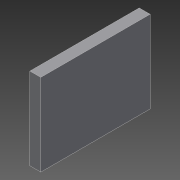
# Autodesk Inventor part: trackballL
Saved by Autodesk Inventor 2018 (Build 220112000, 112)
## iProperties
Created: 2018-06-15
Part Number: trackballL
Material: 一般
Document SubType Name: Sheet Metal
Designer: NaMACHAN
Density: 1 g/cm^3
Sheet Metal Rule: Default
Appearance: 既定
Author: NaMACHAN
Autodesk Inventor part; units mm, degrees
ref_plane "YZ Plane" through (0, 0, 0) normal (1, 0, 0) x (0, 1, 0)
ref_plane "XZ Plane" through (0, 0, 0) normal (0, 1, 0) x (-1, 0, 0)
ref_plane "XY Plane" through (0, 0, 0) normal (0, 0, 1) x (1, 0, 0)
sketch "スケッチ1" plane through (0, 0, 0) normal (1, 0, 0) x (0, 1, 0)
  line L0 (-10, -10) -> (10, -10)
  line L1 (10, -10) -> (10, 10)
  line L2 (10, 10) -> (-10, 10)
  line L3 (-10, 10) -> (-10, -10)
  line L4 (-10, -10) -> (10, 10) construction
  line L5 (10, -10) -> (-10, 10) construction
  point P0 (0, 0)
  dimension "d0" = 20
  dimension "d1" = 20
  measures "d0" distance of L2.end L1.end
  measures "d1" distance of L1.end L0.end
extrude "プレート1" add sketch "スケッチ1" along normal blind 2
sketch "スケッチ2" plane through (4, 12, 10) normal (0, 1, 0) x (-1, 0, 0)
  line L0 (0, -20) -> (0, 0)
  line L1 (0, 0) -> (-21, 0)
  line L2 (-21, 0) -> (-21, -20)
  line L3 (-21, -20) -> (0, -20)
  constraints: 6 end point, 1 horizontal, 1 perpendicular, 1 vertical
edge flange "フランジ1" height 25 angle 90 thickness 2 bend radius 2 thickness toward (0, 1, 0) relief straight relief width 2 relief depth 1 edges at (2, 10, 0) wall of the first edge with corners at (4, 12, -10) (4, 12, 10) (25, 12, 10) (25, 12, -10)
bend "曲げ1"
corner "コーナー1"
sketch "スケッチ3" plane through (0, 0, 0) normal (-1, 0, 0) x (0, 0, 1)
  line L0 (-7.5, 6) -> (-7.5, -6)
  arc A0 (-7.5, -6) -> (-4.5, -6) centre (-6, -6) ccw
  line L1 (-4.5, -6) -> (-4.5, 6)
  arc A1 (-4.5, 6) -> (-7.5, 6) centre (-6, 6) ccw
  line L2 (4.5, 6) -> (4.5, -6)
  arc A2 (4.5, -6) -> (7.5, -6) centre (6, -6) ccw
  line L3 (7.5, -6) -> (7.5, 6)
  arc A3 (7.5, 6) -> (4.5, 6) centre (6, 6) ccw
  line L4 (-10, -10) -> (-10, 10) projected
  line L5 (10, 10) -> (10, -10) projected
  line L6 (10, -10) -> (-10, -10) projected
  line L7 (-10, 10) -> (10, 10) projected
  point P0 (0, 0)
  dimension "d13" = 4
  dimension "d14" = 4
  dimension "d15" = 1.5
  dimension "d16" = 1.5
  dimension "d17" = 4
  dimension "d18" = 4
  dimension "d19" = 4
  dimension "d20" = 4
  constraints: 8 end point, 8 point on circle, 8 tangent, 4 centre point, 2 parallel, 2 vertical
  measures "d13" distance from line of L4 A1.centre
  measures "d14" distance from line of L5 A3.centre
  measures "d15" radius of A1
  measures "d16" radius of A3
  measures "d17" distance from line of L6 A0.centre
  measures "d18" distance from line of L7 A1.centre
  measures "d19" distance from line of L7 A3.centre
  measures "d20" distance from line of A2.centre L6
extrude "押し出し1" cut sketch "スケッチ3" against normal blind 10 contours A1 L1 A0 L0 | A3 L3 A2 L2
equation "\"d2\" = Thickness"
equation "\"d3\" = BendReliefWidth"
equation "\"d4\" = BendReliefDepth"
equation "\"d5\" = MinimumRemnant"
equation "\"d6\" = TransitionRadius"
equation "\"d9\" = BendRadius"
equation "\"d10\" = CornerReliefSize"
equation "\"d11\" = GapSize"
equation "\"d12\" = JacobiRadiusSize"
equation "\"BendRadius\" = Thickness"
equation "\"BendReliefWidth\" = Thickness"
equation "\"BendReliefDepth\" = 0.5 * Thickness"
equation "\"CornerReliefSize\" = 4 * Thickness"
equation "\"MinimumRemnant\" = 2 * Thickness"
equation "\"TransitionRadius\" = BendRadius"
equation "\"JacobiRadiusSize\" = Thickness"
equation "\"GapSize\" = Thickness"
equation "\"Thickness\" = 2"
